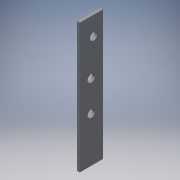
# Autodesk Inventor part: Gear wall motor side
Saved by Autodesk Inventor 2017 (Build 210142000, 142)
## iProperties
Created: 2017-11-21
Part Number: Gear wall motor side
Material: Generic
Document SubType Name: Modeling
Designer: Shlomee
Density: 1 g/cm^3
Appearance: Default
Author: Shlomee
Autodesk Inventor part; units mm, degrees
ref_plane "YZ Plane" through (0, 0, 0) normal (1, 0, 0) x (0, 1, 0)
ref_plane "XZ Plane" through (0, 0, 0) normal (0, 1, 0) x (-1, 0, 0)
ref_plane "XY Plane" through (0, 0, 0) normal (0, 0, 1) x (1, 0, 0)
sketch "Sketch1" plane through (0, 0, 0) normal (0, 0, 1) x (1, 0, 0)
  line L0 (-1.1274, 1.6306) -> (0.8726, 1.6306)
  line L1 (0.8726, 1.6306) -> (0.8726, -14.3694)
  line L2 (0.8726, -14.3694) -> (-1.1274, -14.3694)
  line L3 (-1.1274, -14.3694) -> (-1.1274, 1.6306)
  point P0 (0, 0)
  dimension "d0" = 2
  dimension "d1" = 16
  constraints: 8 end point, 2 parallel, 1 horizontal, 1 perpendicular
  measures "d0" distance of L0.start L0.end
  measures "d1" distance of L0.end L1.end
extrude "Extrusion1" add sketch "Sketch1" along normal blind 89
sketch "Sketch3" plane through (-1.1274, -14.3694, 0) normal (-1, 0, 0) x (0, 0, 1)
  circle A0 centre (31, 7.8652) radius 2.5
  circle A1 centre (52, 7.8652) radius 2.5
  circle A2 centre (76.1354, 9.5069) radius 2.5
  point P0 (0, 14.3694)
  constraints: 3 centre point, 6 other
extrude "Extrusion3" cut sketch "Sketch3" against normal blind 10
body "Solid1"
